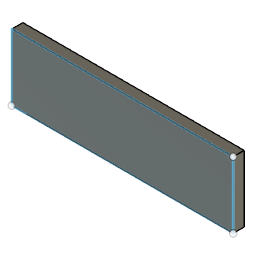
DD-fixation-v6 (Autodesk Fusion 360 design; units mm, degrees)
part number: 2025-12-22-09-38-26-040
Autodesk Fusion 360 part; units mm, degrees
sketch "Esquisse1" plane through (0, 0, 0) normal (0, 1, 0) x (1, 0, 0)
  line L0 (-10, 6) -> (30, 6)
  line L1 (30, 6) -> (30, -6)
  line L2 (30, -6) -> (-10, -6)
  line L3 (-10, -6) -> (-10, 6)
  line L4 (-10, 6) -> (-10, -6)
  line L5 (30, -6) -> (30, 6)
  line L6 (-7.5, 6) -> (-10, 6)
  line L7 (-10, 6) -> (-10, -6)
  line L8 (30, 6) -> (30, -6)
  constraint horizontal L0
  constraint vertical L1
  constraint horizontal L2
  constraint vertical L3
  constraint vertical L4
  constraint vertical L5
  constraint coincident L0 L1.start
  constraint horizontal L6
  constraint vertical L7
  constraint coincident L0 L6.start
  constraint vertical L8
extrude "Extrusion5" add sketch "Esquisse1" along normal blind 2
